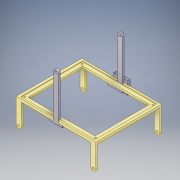
# Autodesk Inventor part: ControllerPCBHolder
Saved by Autodesk Inventor 2019.1 (Build 231200000, 200)
## iProperties
Created: 2018-09-15
Part Number: ControllerPCBHolder
Material: Generisch
Document SubType Name: Modeling
Designer: JochenAlt
Density: 1 g/cm^3
Appearance: Nylon 6
Author: JochenAlt
Autodesk Inventor part; units mm, degrees
ref_plane "YZ Plane" through (0, 0, 0) normal (1, 0, 0) x (0, 1, 0)
ref_plane "XZ Plane" through (0, 0, 0) normal (0, 1, 0) x (-1, 0, 0)
ref_plane "XY Plane" through (0, 0, 0) normal (0, 0, 1) x (1, 0, 0)
sketch "Skizze1" plane through (0, 0, 0) normal (0, 0, 1) x (1, 0, 0)
  line L0 (-60, 50) -> (60, 50)
  line L1 (60, 50) -> (60, -50)
  line L2 (60, -50) -> (-60, -50)
  line L3 (-60, -50) -> (-60, 50)
  line L4 (0, 70) -> (0, -70) construction
  line L5 (-84, 0) -> (84, 0) construction
  line L6 (-54, 44) -> (54, 44)
  line L7 (54, 44) -> (54, -44)
  line L8 (54, -44) -> (-54, -44)
  line L9 (-54, -44) -> (-54, 44)
  line L10 (-57.15, 46.36) -> (57.15, 46.36) construction
  line L11 (57.15, 46.36) -> (57.15, -46.36) construction
  line L12 (57.15, -46.36) -> (-57.15, -46.36) construction
  line L13 (-57.15, -46.36) -> (-57.15, 46.36) construction
  circle A0 centre (-57.15, 46.36) radius 1.25
  circle A1 centre (57.15, 46.36) radius 1.25
  circle A2 centre (-57.15, -46.36) radius 1.25
  circle A3 centre (57.15, -46.36) radius 1.25
  point P0 (0, 0)
  dimension "d0" = 120
  dimension "d1" = 100
  dimension "d4" = 6
  dimension "d5" = 6
  dimension "d6" = 2.5
  dimension "d7" = 114.3
  dimension "d8" = 92.72
  constraints: 24 end point, 6 parallel, 4 centre point, 4 coincident, 3 equal radius, 3 horizontal, 3 perpendicular, 6 other
  measures "d0" distance of L0.start L0.end
  measures "d1" distance of L0.end L1.end
  measures "d4" distance between parallel lines of L6 L0
  measures "d5" distance between parallel lines of L9 L3
  measures "d6" diameter of A0
  measures "d7" distance of L11.end L12.end
  measures "d8" distance of L10.end L11.end
extrude "Extrusion2" add sketch "Skizze1" along normal blind 3
sketch "Skizze2" plane through (0, 0, 0) normal (0, 1, 0) x (-1, 0, 0)
  arc A0 (56.1888, -34.75) -> (64.1888, -34.75) centre (60.1888, -34.75) ccw
  arc A1 (-64.1888, -34.75) -> (-56.1888, -34.75) centre (-60.1888, -34.75) ccw
  line L0 (0, -39.654) -> (0, 10.109) construction
  line L1 (-96.0958, 0) -> (90.9223, 0) construction
  circle A2 centre (60.1888, -34.75) radius 1.75
  circle A3 centre (-60.1888, -34.75) radius 1.75
  line L2 (64.1888, -34.75) -> (64.1888, 3)
  line L3 (56.1888, -34.75) -> (56.1888, 3)
  line L4 (-56.1888, -34.75) -> (-56.1888, 3)
  line L5 (-64.1888, -34.75) -> (-64.1888, 3)
  line L6 (-60, 3) -> (60, 3) construction
  line L7 (64.1888, 3) -> (56.1888, 3)
  line L8 (-64.1888, 3) -> (-56.1888, 3)
  circle A4 centre (0, 69.5) radius 1.75
  arc A5 (4, 69.5) -> (-4, 69.5) centre (0, 69.5) ccw
  line L9 (60.1888, -34.75) -> (0, 69.5) construction
  line L10 (4, 69.5) -> (4, 0)
  line L11 (4, 0) -> (-4, 0)
  line L12 (-4, 0) -> (-4, 69.5)
  line L13 (60, 0) -> (-60, 0) projected
  circle A6 centre (0, 0) radius 69.5 construction
  line L14 (60.1888, -34.75) -> (-60.1888, -34.75) construction
  line L15 (0, 69.5) -> (-60.1888, -34.75) construction
  line L16 (-4.15, -1) -> (-4.15, 4)
  line L17 (-4.15, 4) -> (4.15, 4)
  line L18 (4.15, 4) -> (4.15, -1)
  line L19 (54, 3) -> (-54, 3) construction
  line L20 (4.15, -1) -> (-4.15, -1)
  dimension "d12" = 3.5
  dimension "d22" = 69.5
  dimension "d23" = 4
  dimension "d42" = 0.15
  dimension "d43" = 1
  dimension "d44" = 1
  constraints: 32 end point, 8 point on circle, 7 centre point, 7 point on line, 6 tangent, 5 vertical, 4 coincident, 4 equal radius, 3 equal length, 3 horizontal, 1 collinear, 1 parallel, 1 perpendicular, 2 other
  measures "d12" diameter of A2
  measures "d22" radius of A6
  measures "d23" radius of A0
  measures "d42" distance between parallel lines of L16 L12
  measures "d43" distance between parallel lines of L11 L20
  measures "d44" distance between parallel lines of L19 L17
extrude "Extrusion3" add sketch "Skizze2" along normal blind 3 from surface at 50 contours L3 L7 L2 A0 | L5 L8 L4 A1
extrude "Extrusion4" add sketch "Skizze2" against normal blind 3 from surface at -50 contours L3 L7 L2 A0 | L5 L8 L4 A1
sketch "Skizze4" plane through (0, 0, 0) normal (0, 0, 1) x (1, 0, 0)
  line L0 (-64.1888, 53) -> (-64.1888, 50) projected
  line L1 (56.1888, -53) -> (64.1888, -53) projected
  line L2 (-64.1888, 53) -> (64.1888, 53)
  line L3 (64.1888, 53) -> (64.1888, -53)
  line L4 (64.1888, -53) -> (-64.1888, -53)
  line L5 (-64.1888, -53) -> (-64.1888, 53)
  line L6 (60, -50) -> (60, 50) projected
  line L7 (60, -50) -> (-59.9877, -50)
  line L8 (-59.9877, -50) -> (-59.9877, 50)
  line L9 (-59.9877, 50) -> (60, 50)
  line L10 (60, 50) -> (60, -50)
  point P0 (0, 0)
  constraints: 16 end point, 4 parallel, 2 horizontal, 2 perpendicular
extrude "Extrusion5" add sketch "Skizze4" along normal blind 4
extrude "Extrusion7" cut sketch "Skizze2" along normal up to surface (3 mm away) from surface at -53 contours L17 L18 L13 L10 | L10 L11 L12 L17 | L12 L13 L16 L17 | L13 L18 L20 L16 L11
extrude "Extrusion8" cut sketch "Skizze2" against normal up to surface (3 mm away) from surface at 53 contours L17 L18 L13 L10 | L10 L11 L12 L17 | L12 L13 L16 L17 | L13 L18 L20 L16 L11
sketch "Skizze5" plane through (0, 0, 0) normal (0, 1, 0) x (-1, 0, 0)
  point P0 (0, 0)
sketch "Skizze6" plane through (-56.1888, 53, 0) normal (0, -1, 0) x (1, 0, 0)
  line L0 (-33.6755, 0) -> (146.053, 0) construction
  line L1 (56.1888, 16.75) -> (56.1888, -48) construction
  line L2 (45.1888, 7.5) -> (64.1888, 7.5)
  line L3 (64.1888, 7.5) -> (64.1888, -8.5)
  line L4 (64.1888, -8.5) -> (45.1888, -8.5)
  line L5 (45.1888, -8.5) -> (45.1888, 7.5)
  line L6 (112.3775, 0) -> (0, 0) projected
  circle A0 centre (47.6888, -6) radius 1.75
  circle A1 centre (61.6888, -6) radius 1.75
  line L7 (61.6888, -6) -> (47.6888, -6) construction
  line L8 (54.6888, 7.5) -> (54.6888, -8.5) construction
  line L9 (43.1888, -10.5) -> (66.1888, -10.5)
  line L10 (66.1888, -10.5) -> (66.1888, 9.5)
  line L11 (66.1888, 9.5) -> (43.1888, 9.5)
  line L12 (43.1888, 9.5) -> (43.1888, -10.5)
  point P0 (56.1888, 0)
  point P1 (56.1888, 0)
  point P2 (56.1888, 0)
  dimension "d24" = 19
  dimension "d25" = 16
  dimension "d29" = 7.5
  dimension "d30" = 3.5
  dimension "d31" = 2.5
  dimension "d32" = 14
  dimension "d33" = 8
  dimension "d48" = 2
  constraints: 20 end point, 4 parallel, 3 midpoint, 3 perpendicular, 2 centre point, 2 horizontal, 1 coincident, 1 equal radius, 1 symmetric about line, 4 other
  measures "d24" distance of L3.end L4.end
  measures "d25" distance of L2.end L3.end
  measures "d29" distance from line of L2 point (56.189, 0)
  measures "d30" diameter of A0
  measures "d31" distance from line of L4 L7.start
  measures "d32" distance of L7.start L7.end
  measures "d33" distance between parallel lines of L3 L1
  measures "d48" distance between parallel lines of L4 L9
extrude "Extrusion6" add sketch "Skizze2" against normal up to surface (3 mm away) from surface at -50 separate body contours L10 L17 L12 A5 | L10 L11 L12 L17
extrude "Extrusion9" add sketch "Skizze2" against normal up to surface (3 mm away) from surface at 53 contours L10 L17 L12 A5 | L10 L11 L12 L17 bodies 2
sketch "Skizze7" plane through (4, -53, 0) normal (0, 0, -1) x (-1, 0, 0)
  line L0 (8.15, 0) -> (60.1888, 0) construction
  line L1 (17, 0) -> (14, 0)
  line L2 (-6, 0) -> (-6, 9)
  line L3 (-6, 9) -> (14, 9)
  line L4 (17, 9) -> (17, 0)
  line L5 (58, 9) -> (-50, 9) construction
  line L6 (17, 106) -> (-6, 106)
  line L7 (-6, 106) -> (-6, 97)
  line L8 (-6, 97) -> (17, 97)
  line L9 (17, 97) -> (17, 106)
  line L10 (58, 97) -> (-50, 97) projected
  line L11 (-60.1888, 106) -> (-0.15, 106) projected
  line L12 (8, 3) -> (8, 0) construction
  line L13 (0, 3) -> (0, 0) construction
  line L14 (2.25, 3) -> (5.75, 3) construction
  line L15 (2.25, 0) -> (5.75, 0) construction
  line L16 (8.15, 3) -> (-0.15, 3) construction
  line L17 (4, 3) -> (4, 0) construction
  line L18 (8, 0) -> (0, 0) construction
  line L19 (14, 9) -> (14, 0)
  line L20 (14, 9) -> (17, 9)
  line L21 (14, 0) -> (-6, 0)
  point P0 (4, 53)
  dimension "d45" = 23
  dimension "d51" = 10
  constraints: 24 end point, 7 parallel, 4 point on line, 3 horizontal, 3 perpendicular, 2 collinear, 2 midpoint, 1 other
  measures "d45" distance between parallel lines of L2 L4
  measures "d51" distance between parallel lines of L17 L2
extrude "Extrusion10" add sketch "Skizze7" along normal blind 3 contours L9 L8 L7 L6 bodies 2
extrude "Extrusion12" add sketch "Skizze7" along normal blind 3 contours L21 L2 L3 L19 bodies 2
extrude "Extrusion11" add sketch "Skizze6" against normal blind 4 bodies 2
equation "\"d5\" = d4"
equation "\"d44\" = d43"
